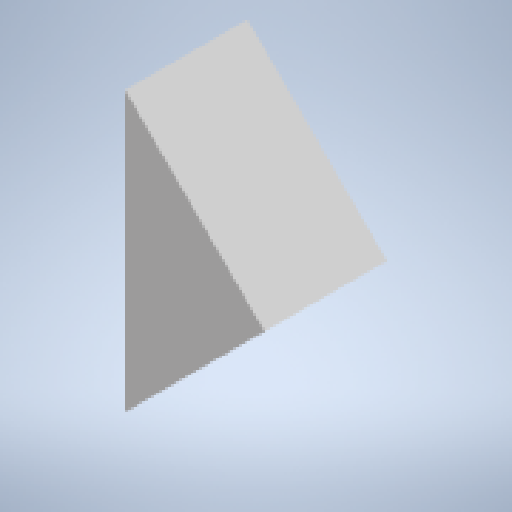
# Autodesk Inventor part: Holder
Saved by Autodesk Inventor 2025.2 (Build 292293000, 293)
## iProperties
Created: 2025-07-25
Part Number: Holder
Material: Generic
Document SubType Name: Modeling
Designer: arbaz
Density: 1 g/cm^3
Appearance: Default
Author: arbaz
Autodesk Inventor part; units mm, degrees
ref_plane "YZ Plane" through (0, 0, 0) normal (1, 0, 0) x (0, 1, 0)
ref_plane "XZ Plane" through (0, 0, 0) normal (0, 1, 0) x (-1, 0, 0)
ref_plane "XY Plane" through (0, 0, 0) normal (0, 0, 1) x (1, 0, 0)
sketch "Sketch1" plane through (0, 0, 0) normal (0, 0, 1) x (1, 0, 0)
  arc A0 (35.4437, -2.2451) -> (35.4437, 2.2451) centre (33.1987, 0) ccw projected
  line L0 (35.4437, 2.2451) -> (-34.1533, 71.842) projected
  line L1 (-34.1533, 71.842) -> (-37.6888, 68.3065) projected
  line L2 (-37.6888, 68.3065) -> (30.6177, 0) projected
  line L3 (30.6177, 0) -> (-37.6888, -68.3065) projected
  line L4 (-37.6888, -68.3065) -> (-34.1533, -71.842) projected
  line L5 (-34.1533, -71.842) -> (35.4437, -2.2451) projected
  line L6 (-37.6888, 68.3065) -> (-37.6888, -68.3065)
  line L7 (-37.6888, 68.3065) -> (30.6177, 0)
  line L8 (-37.6888, -68.3065) -> (30.6177, 0)
  point P0 (0, 0)
  constraints: 6 end point, 1 collinear, 1 vertical
extrude "Extrusion1" add sketch "Sketch1" against normal blind 59.9948 contours L6 L2 L3
sketch "Sketch2" plane through (30.6177, 0, -59.9948) normal (0.7071068, 0.7071068, 0) x (-0.7071068, 0.7071068, 0)
  line L0 (0, 59.9948) -> (96.6, 59.9948) projected
  line L1 (0, 59.9948) -> (0, 0) projected
  line L2 (96.6, 0) -> (0, 0) projected
  line L3 (96.6, 59.9948) -> (96.6, 0) projected
  line L4 (3.85, 55.3974) -> (92.75, 55.3974)
  line L5 (92.75, 55.3974) -> (92.75, 4.5974)
  line L6 (92.75, 4.5974) -> (3.85, 4.5974)
  line L7 (3.85, 4.5974) -> (3.85, 55.3974)
  line L8 (3.85, 55.3974) -> (92.75, 4.5974) construction
  line L9 (92.75, 55.3974) -> (3.85, 4.5974) construction
  point P0 (21.65, 59.9948)
  point P1 (48.3, 29.9974)
  dimension "d2" = 88.9
  dimension "d3" = 50.8
  constraints: 12 end point, 2 midpoint, 2 parallel, 1 horizontal, 1 perpendicular
  measures "d2" distance of L5.end L6.end
  measures "d3" distance of L4.end L5.end
extrude "Extrusion2" cut sketch "Sketch2" against normal blind 59.9948 contours L4 L5 L6 L7
sketch "Sketch3" plane through (-37.6888, -68.3065, 0) normal (0.7071068, -0.7071068, 0) x (-0.7071068, -0.7071068, 0)
  line L0 (-96.6, 4.5974) -> (-36.6052, 4.5974) projected
  line L1 (-96.6, 55.3974) -> (-36.6052, 55.3974) projected
  line L2 (-92.75, 55.3974) -> (-92.75, 4.5974) projected
  line L3 (-92.75, 4.5974) -> (-3.85, 4.5974)
  line L4 (-3.85, 4.5974) -> (-3.85, 55.3974)
  line L5 (-3.85, 55.3974) -> (-92.75, 55.3974)
  line L6 (-92.75, 55.3974) -> (-92.75, 4.5974)
  point P0 (-74.95, 0)
  point P1 (-36.6052, 55.3974)
  point P2 (-36.6052, 4.5974)
  dimension "d6" = 88.9
  constraints: 8 end point, 2 parallel, 1 horizontal, 1 perpendicular
  measures "d6" distance of L5.end L4.end
extrude "Extrusion3" cut sketch "Sketch3" against normal blind 59.9948
sketch "Sketch4" plane through (30.6177, 0, -59.9948) normal (0.7071068, 0.7071068, 0) x (-0.7071068, 0.7071068, 0)
  line L0 (0, 59.9948) -> (96.6, 59.9948) projected
  line L1 (96.6, 0) -> (0, 0) projected
  line L2 (39.5599, 59.9948) -> (52.2599, 59.9948)
  line L3 (52.2599, 59.9948) -> (52.2599, 0)
  line L4 (52.2599, 0) -> (39.5599, 0)
  line L5 (39.5599, 0) -> (39.5599, 59.9948)
  line L6 (92.75, 55.3974) -> (92.75, 4.5974) projected
  line L7 (92.75, 4.5974) -> (3.85, 4.5974) projected
  line L8 (3.85, 4.5974) -> (3.85, 55.3974) projected
  line L9 (3.85, 55.3974) -> (92.75, 55.3974) projected
  line L10 (0, 59.9948) -> (96.6, 59.9948) projected
  line L11 (0, 59.9948) -> (0, 0) projected
  line L12 (96.6, 0) -> (0, 0) projected
  line L13 (96.6, 59.9948) -> (96.6, 0) projected
  point P0 (21.65, 59.9948)
  point P1 (52.2599, 55.3974)
  point P2 (39.5599, 55.3974)
  point P3 (39.5599, 4.5974)
  point P4 (52.2599, 4.5974)
  dimension "d9" = 12.7
  constraints: 8 end point, 2 parallel, 2 point on line, 1 horizontal, 1 perpendicular
  measures "d9" distance of L3.end L4.end
extrude "Extrusion4" add sketch "Sketch4" against normal blind 3 contours L9 L3 L7 L5
sketch "Sketch5" plane through (-37.6888, -68.3065, 0) normal (0.7071068, -0.7071068, 0) x (-0.7071068, -0.7071068, 0)
  line L0 (-3.85, 4.5974) -> (-92.75, 4.5974) projected
  line L1 (-92.75, 55.3974) -> (-3.85, 55.3974) projected
  line L2 (-40.0361, 4.5974) -> (-58.8269, 4.5974)
  line L3 (-58.8269, 4.5974) -> (-58.8269, 55.3974)
  line L4 (-58.8269, 55.3974) -> (-40.0361, 55.3974)
  line L5 (-40.0361, 55.3974) -> (-40.0361, 4.5974)
  point P0 (-74.95, 0)
  point P1 (-40.0361, 55.3974)
  constraints: 8 end point, 2 parallel, 2 point on line, 1 horizontal, 1 perpendicular
extrude "Extrusion5" add sketch "Sketch5" against normal blind 3
sketch "Sketch6" plane through (-37.6888, -68.3065, 0) normal (-1, 0, 0) x (0, 0, 1)
  line L0 (0, 136.613) -> (0, 0) projected
  line L1 (0, 136.613) -> (-59.9948, 136.613) projected
  line L2 (-59.9948, 0) -> (-59.9948, 136.613) projected
  line L3 (0, 0) -> (-59.9948, 0) projected
  line L4 (-4.5974, 131.1683) -> (-4.5974, 5.4447) projected
  line L5 (-4.5974, 5.4447) -> (-55.3974, 5.4447) projected
  line L6 (-55.3974, 5.4447) -> (-55.3974, 131.1683) projected
  line L7 (-55.3974, 131.1683) -> (-4.5974, 131.1683) projected
  point P0 (0, 68.3065)
extrude "Extrusion6" add sketch "Sketch6" against normal blind 3 contours L4 L5 L6 L7
sketch "Sketch7" plane through (0, 0, -59.9948) normal (0, 0, -1) x (-1, 0, 0)
  line L0 (37.6888, 68.3065) -> (-30.6177, 0) projected
  line L1 (37.6888, 68.3065) -> (37.6888, 73.3065)
  line L2 (37.6888, 73.3065) -> (-37.195, -1.5773)
  line L3 (37.6888, -68.3065) -> (37.6888, 68.3065) projected
  line L4 (37.6888, -68.3065) -> (37.6888, -73.3065)
  line L5 (37.6888, -73.3065) -> (-46.9966, 11.3789)
  point P0 (0, 0)
  point P1 (-35.6177, 0)
  dimension "d16" = 5
  dimension "d17" = 45
  dimension "d18" = 5
  constraints: 8 end point, 2 vertical
  measures "d16" distance of L0.start L1.end
  measures "d17" angle of L2 L1
  measures "d18" distance of L3.start L4.end
extrude "Extrusion7" add sketch "Sketch7" along normal blind 3
sketch "Sketch8" plane through (0, 0, 0) normal (0, 0, 1) x (1, 0, 0)
  line L0 (-37.6888, -68.3065) -> (30.6177, 0) projected
  line L1 (30.6177, 0) -> (-37.6888, 68.3065) projected
  line L2 (-37.6888, 68.3065) -> (-37.6888, -68.3065) projected
  line L3 (-37.6888, 73.3065) -> (35.6177, 0) projected
  line L4 (-37.6888, 68.3065) -> (-37.6888, 73.3065) projected
  line L5 (-37.6888, -73.3065) -> (-37.6888, -68.3065) projected
  line L6 (35.6177, 0) -> (-37.6888, -73.3065) projected
  point P0 (0, 0)
extrude "Extrusion8" add sketch "Sketch8" along normal blind 3
sketch "Sketch9" plane through (0, 0, 3) normal (0, 0, 1) x (1, 0, 0)
  circle A0 centre (-11.7105, 0) radius 19.05
  point P0 (0, 0)
  dimension "d23" = 38.1
  constraints: 1 centre point
  measures "d23" diameter of A0
extrude "Extrusion9" add sketch "Sketch9" along normal blind 38.1
sketch "Sketch10" plane through (-11.7105, 0, 41.1) normal (0, 0, 1) x (1, 0, 0)
  line L0 (19.05, -19.05) -> (-19.05, -19.05)
  line L1 (-19.05, -19.05) -> (-19.05, 19.05)
  line L2 (-19.05, 19.05) -> (19.05, 19.05)
  line L3 (19.05, 19.05) -> (19.05, -19.05)
  line L4 (19.05, -19.05) -> (-19.05, 19.05) construction
  line L5 (-19.05, -19.05) -> (19.05, 19.05) construction
  point P0 (11.7105, 0)
  point P1 (0, 0)
  dimension "d26" = 38.1
  dimension "d27" = 38.1
  constraints: 12 end point, 2 midpoint, 2 parallel, 1 horizontal, 1 perpendicular
  measures "d26" distance of L1.end L2.end
  measures "d27" distance of L0.end L1.end
extrude "Extrusion10" add sketch "Sketch10" along normal blind 38.1
sketch "Sketch11" plane through (7.3395, -19.05, 41.1) normal (1, 0, 0) x (0, 0, -1)
  line L0 (0, 0) -> (0, 19.05) projected
  line L1 (0, 19.05) -> (0, 38.1) projected
  line L2 (0, 38.1) -> (-38.1, 38.1) projected
  line L3 (-38.1, 0) -> (-38.1, 38.1) projected
  line L4 (0, 0) -> (-38.1, 0) projected
  circle A0 centre (-19.05, 19.05) radius 15.24
  point P0 (41.1, 19.05)
  dimension "d30" = 30.48
  constraints: 1 centre point
  measures "d30" diameter of A0
extrude "Extrusion11" cut sketch "Sketch11" against normal blind 50.8 contours A0
fillet "Fillet1" radius 12.7 2 edges at (-11.7105, -19.05, 79.2) (-11.7105, 19.05, 79.2)
fillet "Fillet2" radius 12.7 4 edges at (-2.1855, 19.05, 41.1) (-21.2355, 19.05, 41.1) (-21.2355, -19.05, 41.1) (-2.1855, -19.05, 41.1)
body "Solid1"
